Autodesk Inventor part; units mm, degrees
(part 3 of 6)
  arc A229 (-128.6396, 107.7295) -> (-129.027, 107.8036) centre (-130.0365, 101.4759) ccw projected
  arc A230 (-128.1665, 107.6078) -> (-128.6396, 107.7295) centre (-130.2936, 100.3247) ccw projected
  arc A231 (-128.1196, 107.2111) -> (-128.1665, 107.6078) centre (-148.5, 105) ccw projected
  arc A232 (-128.5511, 106.9822) -> (-128.1196, 107.2111) centre (-131.8881, 113.7963) ccw projected
  arc A233 (-128.9105, 106.8197) -> (-128.5511, 106.9822) centre (-131.3693, 112.7369) ccw projected
  arc A234 (-129.2005, 106.7091) -> (-128.9105, 106.8197) centre (-130.9335, 111.6881) ccw projected
  arc A235 (-129.1708, 106.331) -> (-129.2005, 106.7091) centre (-148.5, 105) ccw projected
  arc A236 (-128.867, 106.2671) -> (-129.1708, 106.331) centre (-130.1035, 101.1423) ccw projected
  arc A237 (-128.4867, 106.1629) -> (-128.867, 106.2671) centre (-130.3699, 100.0382) ccw projected
  arc A238 (-128.0246, 106.0044) -> (-128.4867, 106.1629) centre (-130.7166, 98.9106) ccw projected
  arc A239 (-128.0089, 105.6052) -> (-128.0246, 106.0044) centre (-148.5, 105) ccw projected
  arc A240 (-128.4571, 105.4109) -> (-128.0089, 105.6052) centre (-131.2492, 112.4658) ccw projected
  arc A241 (-128.8281, 105.2771) -> (-128.4571, 105.4109) centre (-130.8151, 111.369) ccw projected
  arc A242 (-129.1259, 105.1896) -> (-128.8281, 105.2771) centre (-130.4629, 110.2892) ccw projected
  arc A243 (-129.1259, 104.8104) -> (-129.1259, 105.1896) centre (-148.5, 105) ccw projected
  arc A244 (-128.8281, 104.7229) -> (-129.1259, 104.8104) centre (-130.4629, 99.7108) ccw projected
  arc A245 (-128.4571, 104.5891) -> (-128.8281, 104.7229) centre (-130.8151, 98.631) ccw projected
  arc A246 (-128.0089, 104.3948) -> (-128.4571, 104.5891) centre (-131.2492, 97.5342) ccw projected
  arc A247 (-128.0246, 103.9956) -> (-128.0089, 104.3948) centre (-148.5, 105) ccw projected
  arc A248 (-128.4867, 103.8371) -> (-128.0246, 103.9956) centre (-130.7166, 111.0894) ccw projected
  arc A249 (-128.867, 103.7329) -> (-128.4867, 103.8371) centre (-130.3699, 109.9618) ccw projected
  arc A250 (-129.1708, 103.669) -> (-128.867, 103.7329) centre (-130.1035, 108.8577) ccw projected
  arc A251 (-129.2005, 103.2909) -> (-129.1708, 103.669) centre (-148.5, 105) ccw projected
  arc A252 (-128.9105, 103.1803) -> (-129.2005, 103.2909) centre (-130.9335, 98.3119) ccw projected
  arc A253 (-128.5511, 103.0178) -> (-128.9105, 103.1803) centre (-131.3693, 97.2631) ccw projected
  arc A254 (-128.1196, 102.7889) -> (-128.5511, 103.0178) centre (-131.8881, 96.2037) ccw projected
  arc A255 (-128.1665, 102.3922) -> (-128.1196, 102.7889) centre (-148.5, 105) ccw projected
  arc A256 (-128.6396, 102.2705) -> (-128.1665, 102.3922) centre (-130.2936, 109.6753) ccw projected
  arc A257 (-129.027, 102.1964) -> (-128.6396, 102.2705) centre (-130.0365, 108.5241) ccw projected
  arc A258 (-129.3348, 102.1565) -> (-129.027, 102.1964) centre (-129.8575, 107.4025) ccw projected
  arc A259 (-129.3941, 101.7819) -> (-129.3348, 102.1565) centre (-148.5, 105) ccw projected
  arc A260 (-129.1137, 101.6489) -> (-129.3941, 101.7819) centre (-131.5124, 96.9543) ccw projected
  arc A261 (-128.7682, 101.4587) -> (-129.1137, 101.6489) centre (-132.0292, 95.9429) ccw projected
  arc A262 (-128.3559, 101.1967) -> (-128.7682, 101.4587) centre (-132.6295, 94.9274) ccw projected
  arc A263 (-128.4338, 100.8049) -> (-128.3559, 101.1967) centre (-148.5, 105) ccw projected
  arc A264 (-128.915, 100.7207) -> (-128.4338, 100.8049) centre (-129.983, 108.2324) ccw projected
  arc A265 (-129.307, 100.6772) -> (-128.915, 100.7207) centre (-129.8169, 107.0646) ccw projected
  arc A266 (-129.617, 100.6616) -> (-129.307, 100.6772) centre (-129.7265, 105.9324) ccw projected
  arc A267 (-129.7055, 100.2928) -> (-129.617, 100.6616) centre (-148.5, 105) ccw projected
  arc A268 (-129.4364, 100.1382) -> (-129.7055, 100.2928) centre (-132.196, 95.6463) ccw projected
  arc A269 (-129.1068, 99.9215) -> (-129.4364, 100.1382) centre (-132.7905, 94.6785) ccw projected
  arc A270 (-128.7164, 99.628) -> (-129.1068, 99.9215) centre (-133.4687, 93.7133) ccw projected
  arc A271 (-128.8248, 99.2435) -> (-128.7164, 99.628) centre (-148.5, 105) ccw projected
  arc A272 (-129.3111, 99.1972) -> (-128.8248, 99.2435) centre (-129.7864, 106.7696) ccw projected
  arc A273 (-129.7053, 99.1846) -> (-129.3111, 99.1972) centre (-129.7125, 105.5924) ccw projected
  arc A274 (-130.0156, 99.1934) -> (-129.7053, 99.1846) centre (-129.7112, 104.4566) ccw projected
  arc A275 (-130.1328, 98.8327) -> (-130.0156, 99.1934) centre (-148.5, 105) ccw projected
  arc A276 (-129.8766, 98.6575) -> (-130.1328, 98.8327) centre (-132.9801, 94.3959) ccw projected
  arc A277 (-129.5651, 98.4156) -> (-129.8766, 98.6575) centre (-133.6488, 93.4778) ccw projected
  arc A278 (-129.1989, 98.0923) -> (-129.5651, 98.4156) centre (-134.4006, 92.5688) ccw projected
  arc A279 (-129.3371, 97.7175) -> (-129.1989, 98.0923) centre (-148.5, 105) ccw projected
  arc A280 (-129.8255, 97.7096) -> (-129.3371, 97.7175) centre (-129.7053, 105.2959) ccw projected
  arc A281 (-130.2195, 97.728) -> (-129.8255, 97.7096) centre (-129.724, 104.1165) ccw projected
  arc A282 (-130.5281, 97.7611) -> (-130.2195, 97.728) centre (-129.8118, 102.9841) ccw projected
  arc A283 (-130.6733, 97.4107) -> (-130.5281, 97.7611) centre (-148.5, 105) ccw projected
  arc A284 (-130.4316, 97.2158) -> (-130.6733, 97.4107) centre (-133.86, 93.2109) ccw projected
  arc A285 (-130.14, 96.9503) -> (-130.4316, 97.2158) centre (-134.5986, 92.3481) ccw projected
  arc A286 (-129.8003, 96.5993) -> (-130.14, 96.9503) centre (-135.4194, 91.5009) ccw projected
  arc A287 (-129.9676, 96.2365) -> (-129.8003, 96.5993) centre (-148.5, 105) ccw projected
  arc A288 (-130.4551, 96.2669) -> (-129.9676, 96.2365) centre (-129.74, 103.8204) ccw projected
  arc A289 (-130.8464, 96.3161) -> (-130.4551, 96.2669) centre (-129.8512, 102.6461) ccw projected
  arc A290 (-131.1515, 96.3733) -> (-130.8464, 96.3161) centre (-130.0276, 101.524) ccw projected
  arc A291 (-131.3237, 96.0354) -> (-131.1515, 96.3733) centre (-148.5, 105) ccw projected
  arc A292 (-131.0981, 95.8222) -> (-131.3237, 96.0354) centre (-134.8301, 92.0986) ccw projected
  arc A293 (-130.8282, 95.5346) -> (-131.0981, 95.8222) centre (-135.6341, 91.2964) ccw projected
  arc A294 (-130.5171, 95.158) -> (-130.8282, 95.5346) centre (-136.5188, 90.5162) ccw projected
  arc A295 (-130.7123, 94.8095) -> (-130.5171, 95.158) centre (-148.5, 105) ccw projected
  arc A296 (-131.1959, 94.878) -> (-130.7123, 94.8095) centre (-129.8904, 102.3522) ccw projected
  arc A297 (-131.5822, 94.9578) -> (-131.1959, 94.878) centre (-130.0933, 101.1901) ccw projected
  arc A298 (-131.8818, 95.0388) -> (-131.5822, 94.9578) centre (-130.3572, 100.0854) ccw projected
  arc A299 (-132.08, 94.7154) -> (-131.8818, 95.0388) centre (-148.5, 105) ccw projected
  arc A300 (-131.8718, 94.4852) -> (-132.08, 94.7154) centre (-135.8844, 91.0659) ccw projected
  arc A301 (-131.6253, 94.1773) -> (-131.8718, 94.4852) centre (-136.7489, 90.3292) ccw projected
  arc A302 (-131.3447, 93.7774) -> (-131.6253, 94.1773) centre (-137.6922, 89.6208) ccw projected
  arc A303 (-131.5666, 93.4453) -> (-131.3447, 93.7774) centre (-148.5, 105) ccw projected
  arc A304 (-132.0434, 93.5515) -> (-131.5666, 93.4453) centre (-130.1555, 100.9002) ccw projected
  arc A305 (-132.4222, 93.6614) -> (-132.0434, 93.5515) centre (-130.449, 99.7577) ccw projected
  arc A306 (-132.7146, 93.7656) -> (-132.4222, 93.6614) centre (-130.7988, 98.6771) ccw projected
  arc A307 (-132.9375, 93.4588) -> (-132.7146, 93.7656) centre (-148.5, 105) ccw projected
  arc A308 (-132.748, 93.2129) -> (-132.9375, 93.4588) centre (-137.0166, 90.119) ccw projected
  arc A309 (-132.5265, 92.8866) -> (-132.748, 93.2129) centre (-137.9362, 89.4524) ccw projected
  arc A310 (-132.2781, 92.466) -> (-132.5265, 92.8866) centre (-138.9321, 88.8202) ccw projected
  arc A311 (-132.5254, 92.1523) -> (-132.2781, 92.466) centre (-148.5, 105) ccw projected
  arc A312 (-132.9924, 92.2957) -> (-132.5254, 92.1523) centre (-130.5337, 99.4736) ccw projected
  arc A313 (-133.3614, 92.4349) -> (-132.9924, 92.2957) centre (-130.9159, 98.3576) ccw projected
  arc A314 (-133.6447, 92.5617) -> (-133.3614, 92.4349) centre (-131.3494, 97.3078) ccw projected
  arc A315 (-133.891, 92.2734) -> (-133.6447, 92.5617) centre (-148.5, 105) ccw projected
  arc A316 (-133.7214, 92.0134) -> (-133.891, 92.2734) centre (-138.2195, 89.2639) ccw projected
  arc A317 (-133.5261, 91.6707) -> (-133.7214, 92.0134) centre (-139.1886, 88.6715) ccw projected
  arc A318 (-133.3115, 91.2319) -> (-133.5261, 91.6707) centre (-140.2311, 88.1194) ccw projected
  arc A319 (-133.5827, 90.9386) -> (-133.3115, 91.2319) centre (-148.5, 105) ccw projected
  arc A320 (-134.037, 91.1181) -> (-133.5827, 90.9386) centre (-131.0227, 98.081) ccw projected
  arc A321 (-134.3939, 91.2859) -> (-134.037, 91.1181) centre (-131.4913, 96.9985) ccw projected
  arc A322 (-134.6664, 91.4345) -> (-134.3939, 91.2859) centre (-132.0058, 95.9859) ccw projected
  arc A323 (-134.9345, 91.1664) -> (-134.6664, 91.4345) centre (-148.5, 105) ccw projected
  arc A324 (-134.7859, 90.8939) -> (-134.9345, 91.1664) centre (-139.4859, 88.5058) ccw projected
  arc A325 (-134.6181, 90.537) -> (-134.7859, 90.8939) centre (-140.4985, 87.9913) ccw projected
  arc A326 (-134.4386, 90.0827) -> (-134.6181, 90.537) centre (-141.581, 87.5227) ccw projected
  arc A327 (-134.7319, 89.8115) -> (-134.4386, 90.0827) centre (-148.5, 105) ccw projected
  arc A328 (-135.1707, 90.0261) -> (-134.7319, 89.8115) centre (-131.6194, 96.7311) ccw projected
  arc A329 (-135.5134, 90.2214) -> (-135.1707, 90.0261) centre (-132.1715, 95.6886) ccw projected
  arc A330 (-135.7734, 90.391) -> (-135.5134, 90.2214) centre (-132.7639, 94.7195) ccw projected
  arc A331 (-136.0617, 90.1447) -> (-135.7734, 90.391) centre (-148.5, 105) ccw projected
  arc A332 (-135.9349, 89.8614) -> (-136.0617, 90.1447) centre (-140.8078, 87.8494) ccw projected
  arc A333 (-135.7957, 89.4924) -> (-135.9349, 89.8614) centre (-141.8576, 87.4159) ccw projected
  arc A334 (-135.6523, 89.0254) -> (-135.7957, 89.4924) centre (-142.9736, 87.0337) ccw projected
  arc A335 (-135.966, 88.7781) -> (-135.6523, 89.0254) centre (-148.5, 105) ccw projected
  arc A336 (-136.3866, 89.0265) -> (-135.966, 88.7781) centre (-132.3202, 95.4321) ccw projected
  arc A337 (-136.7129, 89.248) -> (-136.3866, 89.0265) centre (-132.9524, 94.4362) ccw projected
  arc A338 (-136.9588, 89.4375) -> (-136.7129, 89.248) centre (-133.619, 93.5166) ccw projected
  arc A339 (-137.2656, 89.2146) -> (-136.9588, 89.4375) centre (-148.5, 105) ccw projected
  arc A340 (-137.1614, 88.9222) -> (-137.2656, 89.2146) centre (-142.1771, 87.2988) ccw projected
  arc A341 (-137.0515, 88.5434) -> (-137.1614, 88.9222) centre (-143.2577, 86.949) ccw projected
  arc A342 (-136.9453, 88.0666) -> (-137.0515, 88.5434) centre (-144.4002, 86.6555) ccw projected
  arc A343 (-137.2774, 87.8447) -> (-136.9453, 88.0666) centre (-148.5, 105) ccw projected
  arc A344 (-137.6773, 88.1253) -> (-137.2774, 87.8447) centre (-133.1208, 94.1922) ccw projected
  arc A345 (-137.9852, 88.3718) -> (-137.6773, 88.1253) centre (-133.8292, 93.2489) ccw projected
  arc A346 (-138.2154, 88.58) -> (-137.9852, 88.3718) centre (-134.5659, 92.3844) ccw projected
  arc A347 (-138.5388, 88.3818) -> (-138.2154, 88.58) centre (-148.5, 105) ccw projected
  arc A348 (-138.4578, 88.0822) -> (-138.5388, 88.3818) centre (-143.5854, 86.8572) ccw projected
  arc A349 (-138.378, 87.6959) -> (-138.4578, 88.0822) centre (-144.6901, 86.5933) ccw projected
  arc A350 (-138.3095, 87.2123) -> (-138.378, 87.6959) centre (-145.8522, 86.3904) ccw projected
  arc A351 (-138.658, 87.0171) -> (-138.3095, 87.2123) centre (-148.5, 105) ccw projected
  arc A352 (-139.0346, 87.3282) -> (-138.658, 87.0171) centre (-134.0162, 93.0188) ccw projected
  arc A353 (-139.3222, 87.5981) -> (-139.0346, 87.3282) centre (-134.7964, 92.1341) ccw projected
  arc A354 (-139.5354, 87.8237) -> (-139.3222, 87.5981) centre (-135.5986, 91.3301) ccw projected
  arc A355 (-139.8733, 87.6515) -> (-139.5354, 87.8237) centre (-148.5, 105) ccw projected
  arc A356 (-139.8161, 87.3464) -> (-139.8733, 87.6515) centre (-145.024, 86.5276) ccw projected
  arc A357 (-139.7669, 86.9551) -> (-139.8161, 87.3464) centre (-146.1461, 86.3512) ccw projected
  arc A358 (-139.7365, 86.4676) -> (-139.7669, 86.9551) centre (-147.3204, 86.24) ccw projected
  arc A359 (-140.0993, 86.3003) -> (-139.7365, 86.4676) centre (-148.5, 105) ccw projected
  arc A360 (-140.4503, 86.64) -> (-140.0993, 86.3003) centre (-135.0009, 91.9194) ccw projected
  arc A361 (-140.7158, 86.9316) -> (-140.4503, 86.64) centre (-135.8481, 91.0986) ccw projected
  arc A362 (-140.9107, 87.1733) -> (-140.7158, 86.9316) centre (-136.7109, 90.36) ccw projected
  arc A363 (-141.2611, 87.0281) -> (-140.9107, 87.1733) centre (-148.5, 105) ccw projected
  arc A364 (-141.228, 86.7195) -> (-141.2611, 87.0281) centre (-146.4841, 86.3118) ccw projected
  arc A365 (-141.2096, 86.3255) -> (-141.228, 86.7195) centre (-147.6165, 86.224) ccw projected
  arc A366 (-141.2175, 85.8371) -> (-141.2096, 86.3255) centre (-148.7959, 86.2053) ccw projected
  arc A367 (-141.5923, 85.6989) -> (-141.2175, 85.8371) centre (-148.5, 105) ccw projected
  arc A368 (-141.9156, 86.0651) -> (-141.5923, 85.6989) centre (-136.0688, 90.9006) ccw projected
  arc A369 (-142.1575, 86.3766) -> (-141.9156, 86.0651) centre (-136.9778, 90.1488) ccw projected
  arc A370 (-142.3327, 86.6328) -> (-142.1575, 86.3766) centre (-137.8959, 89.4801) ccw projected
  arc A371 (-142.6934, 86.5156) -> (-142.3327, 86.6328) centre (-148.5, 105) ccw projected
  arc A372 (-142.6846, 86.2053) -> (-142.6934, 86.5156) centre (-147.9566, 86.2112) ccw projected
  arc A373 (-142.6972, 85.8111) -> (-142.6846, 86.2053) centre (-149.0924, 86.2125) ccw projected
  arc A374 (-142.7435, 85.3248) -> (-142.6972, 85.8111) centre (-150.2696, 86.2864) ccw projected
  arc A375 (-143.128, 85.2164) -> (-142.7435, 85.3248) centre (-148.5, 105) ccw projected
  arc A376 (-143.4215, 85.6068) -> (-143.128, 85.2164) centre (-137.2133, 89.9687) ccw projected
  arc A377 (-143.6382, 85.9364) -> (-143.4215, 85.6068) centre (-138.1785, 89.2905) ccw projected
  arc A378 (-143.7928, 86.2055) -> (-143.6382, 85.9364) centre (-139.1463, 88.696) ccw projected
  arc A379 (-144.1616, 86.117) -> (-143.7928, 86.2055) centre (-148.5, 105) ccw projected
  arc A380 (-144.1772, 85.807) -> (-144.1616, 86.117) centre (-149.4324, 86.2265) ccw projected
  arc A381 (-144.2207, 85.415) -> (-144.1772, 85.807) centre (-150.5646, 86.3169) ccw projected
  arc A382 (-144.3049, 84.9338) -> (-144.2207, 85.415) centre (-151.7324, 86.483) ccw projected
  arc A383 (-144.6967, 84.8559) -> (-144.3049, 84.9338) centre (-148.5, 105) ccw projected
  arc A384 (-144.9587, 85.2682) -> (-144.6967, 84.8559) centre (-138.4274, 89.1295) ccw projected
  arc A385 (-145.1489, 85.6137) -> (-144.9587, 85.2682) centre (-139.4429, 88.5292) ccw projected
  arc A386 (-145.2819, 85.8941) -> (-145.1489, 85.6137) centre (-140.4543, 88.0124) ccw projected
  arc A387 (-145.6565, 85.8348) -> (-145.2819, 85.8941) centre (-148.5, 105) ccw projected
  arc A388 (-145.6964, 85.527) -> (-145.6565, 85.8348) centre (-150.9025, 86.3575) ccw projected
  arc A389 (-145.7705, 85.1396) -> (-145.6964, 85.527) centre (-152.0241, 86.5365) ccw projected
  arc A390 (-145.8922, 84.6665) -> (-145.7705, 85.1396) centre (-153.1753, 86.7936) ccw projected
  arc A391 (-146.2889, 84.6196) -> (-145.8922, 84.6665) centre (-148.5, 105) ccw projected
  arc A392 (-146.5178, 85.0511) -> (-146.2889, 84.6196) centre (-139.7037, 88.3881) ccw projected
  arc A393 (-146.6803, 85.4105) -> (-146.5178, 85.0511) centre (-140.7631, 87.8693) ccw projected
  arc A394 (-146.7909, 85.7005) -> (-146.6803, 85.4105) centre (-141.8119, 87.4335) ccw projected
  arc A395 (-147.169, 85.6708) -> (-146.7909, 85.7005) centre (-148.5, 105) ccw projected
  arc A396 (-147.2329, 85.367) -> (-147.169, 85.6708) centre (-152.3577, 86.6035) ccw projected
  arc A397 (-147.3371, 84.9867) -> (-147.2329, 85.367) centre (-153.4618, 86.8699) ccw projected
  arc A398 (-147.4956, 84.5246) -> (-147.3371, 84.9867) centre (-154.5894, 87.2166) ccw projected
  arc A399 (-147.8948, 84.5089) -> (-147.4956, 84.5246) centre (-148.5, 105) ccw projected
  arc A400 (-148.0891, 84.9571) -> (-147.8948, 84.5089) centre (-141.0342, 87.7492) ccw projected
  arc A401 (-148.2229, 85.3281) -> (-148.0891, 84.9571) centre (-142.131, 87.3151) ccw projected
  arc A402 (-148.3104, 85.6259) -> (-148.2229, 85.3281) centre (-143.2108, 86.9629) ccw projected
  arc A403 (-148.6896, 85.6259) -> (-148.3104, 85.6259) centre (-148.5, 105) ccw projected
  arc A404 (-148.7771, 85.3281) -> (-148.6896, 85.6259) centre (-153.7892, 86.9629) ccw projected
  arc A405 (-148.9109, 84.9571) -> (-148.7771, 85.3281) centre (-154.869, 87.3151) ccw projected
  arc A406 (-149.1052, 84.5089) -> (-148.9109, 84.9571) centre (-155.9658, 87.7492) ccw projected
  arc A407 (-149.5044, 84.5246) -> (-149.1052, 84.5089) centre (-148.5, 105) ccw projected
  arc A408 (-149.6629, 84.9867) -> (-149.5044, 84.5246) centre (-142.4106, 87.2166) ccw projected
  arc A409 (-149.7671, 85.367) -> (-149.6629, 84.9867) centre (-143.5382, 86.8699) ccw projected
  arc A410 (-149.831, 85.6708) -> (-149.7671, 85.367) centre (-144.6423, 86.6035) ccw projected
  arc A411 (-150.2091, 85.7005) -> (-149.831, 85.6708) centre (-148.5, 105) ccw projected
  arc A412 (-150.3197, 85.4105) -> (-150.2091, 85.7005) centre (-155.1881, 87.4335) ccw projected
  arc A413 (-150.4822, 85.0511) -> (-150.3197, 85.4105) centre (-156.2369, 87.8693) ccw projected
  arc A414 (-150.7111, 84.6196) -> (-150.4822, 85.0511) centre (-157.2963, 88.3881) ccw projected
  arc A415 (-151.1078, 84.6665) -> (-150.7111, 84.6196) centre (-148.5, 105) ccw projected
  arc A416 (-151.2295, 85.1396) -> (-151.1078, 84.6665) centre (-143.8247, 86.7936) ccw projected
  arc A417 (-151.3036, 85.527) -> (-151.2295, 85.1396) centre (-144.9759, 86.5365) ccw projected
  arc A418 (-151.3435, 85.8348) -> (-151.3036, 85.527) centre (-146.0975, 86.3575) ccw projected
  arc A419 (-151.7181, 85.8941) -> (-151.3435, 85.8348) centre (-148.5, 105) ccw projected
  arc A420 (-151.8511, 85.6137) -> (-151.7181, 85.8941) centre (-156.5457, 88.0124) ccw projected
  arc A421 (-152.0413, 85.2682) -> (-151.8511, 85.6137) centre (-157.5571, 88.5292) ccw projected
  arc A422 (-152.3033, 84.8559) -> (-152.0413, 85.2682) centre (-158.5726, 89.1295) ccw projected
  arc A423 (-152.6951, 84.9338) -> (-152.3033, 84.8559) centre (-148.5, 105) ccw projected
  arc A424 (-152.7793, 85.415) -> (-152.6951, 84.9338) centre (-145.2676, 86.483) ccw projected
  arc A425 (-152.8228, 85.807) -> (-152.7793, 85.415) centre (-146.4354, 86.3169) ccw projected
  arc A426 (-152.8384, 86.117) -> (-152.8228, 85.807) centre (-147.5676, 86.2265) ccw projected
  arc A427 (-153.2072, 86.2055) -> (-152.8384, 86.117) centre (-148.5, 105) ccw projected
  arc A428 (-153.3618, 85.9364) -> (-153.2072, 86.2055) centre (-157.8537, 88.696) ccw projected
  arc A429 (-153.5785, 85.6068) -> (-153.3618, 85.9364) centre (-158.8215, 89.2905) ccw projected
  arc A430 (-153.872, 85.2164) -> (-153.5785, 85.6068) centre (-159.7867, 89.9687) ccw projected
  arc A431 (-154.2565, 85.3248) -> (-153.872, 85.2164) centre (-148.5, 105) ccw projected
  arc A432 (-154.3028, 85.8111) -> (-154.2565, 85.3248) centre (-146.7304, 86.2864) ccw projected
  arc A433 (-154.3154, 86.2053) -> (-154.3028, 85.8111) centre (-147.9076, 86.2125) ccw projected
  arc A434 (-154.3066, 86.5156) -> (-154.3154, 86.2053) centre (-149.0434, 86.2112) ccw projected
  arc A435 (-154.6673, 86.6328) -> (-154.3066, 86.5156) centre (-148.5, 105) ccw projected
  arc A436 (-154.8425, 86.3766) -> (-154.6673, 86.6328) centre (-159.1041, 89.4801) ccw projected
  arc A437 (-155.0844, 86.0651) -> (-154.8425, 86.3766) centre (-160.0222, 90.1488) ccw projected
  arc A438 (-155.4077, 85.6989) -> (-155.0844, 86.0651) centre (-160.9312, 90.9006) ccw projected
  arc A439 (-155.7825, 85.8371) -> (-155.4077, 85.6989) centre (-148.5, 105) ccw projected
  arc A440 (-155.7904, 86.3255) -> (-155.7825, 85.8371) centre (-148.2041, 86.2053) ccw projected
  arc A441 (-155.772, 86.7195) -> (-155.7904, 86.3255) centre (-149.3835, 86.224) ccw projected
  arc A442 (-155.7389, 87.0281) -> (-155.772, 86.7195) centre (-150.5159, 86.3118) ccw projected
  arc A443 (-156.0893, 87.1733) -> (-155.7389, 87.0281) centre (-148.5, 105) ccw projected
  arc A444 (-156.2842, 86.9316) -> (-156.0893, 87.1733) centre (-160.2891, 90.36) ccw projected
  arc A445 (-156.5497, 86.64) -> (-156.2842, 86.9316) centre (-161.1519, 91.0986) ccw projected
  arc A446 (-156.9007, 86.3003) -> (-156.5497, 86.64) centre (-161.9991, 91.9194) ccw projected
  arc A447 (-157.2635, 86.4676) -> (-156.9007, 86.3003) centre (-148.5, 105) ccw projected
  arc A448 (-157.2331, 86.9551) -> (-157.2635, 86.4676) centre (-149.6796, 86.24) ccw projected
  arc A449 (-157.1839, 87.3464) -> (-157.2331, 86.9551) centre (-150.8539, 86.3512) ccw projected
  arc A450 (-157.1267, 87.6515) -> (-157.1839, 87.3464) centre (-151.976, 86.5276) ccw projected
  arc A451 (-157.4646, 87.8237) -> (-157.1267, 87.6515) centre (-148.5, 105) ccw projected
  arc A452 (-157.6778, 87.5981) -> (-157.4646, 87.8237) centre (-161.4014, 91.3301) ccw projected
  arc A453 (-157.9654, 87.3282) -> (-157.6778, 87.5981) centre (-162.2036, 92.1341) ccw projected
  arc A454 (-158.342, 87.0171) -> (-157.9654, 87.3282) centre (-162.9838, 93.0188) ccw projected
  arc A455 (-158.6905, 87.2123) -> (-158.342, 87.0171) centre (-148.5, 105) ccw projected
  arc A456 (-158.622, 87.6959) -> (-158.6905, 87.2123) centre (-151.1478, 86.3904) ccw projected
  arc A457 (-158.5422, 88.0822) -> (-158.622, 87.6959) centre (-152.3099, 86.5933) ccw projected
  arc A458 (-158.4612, 88.3818) -> (-158.5422, 88.0822) centre (-153.4146, 86.8572) ccw projected
  arc A459 (-158.7846, 88.58) -> (-158.4612, 88.3818) centre (-148.5, 105) ccw projected
  arc A460 (-159.0148, 88.3718) -> (-158.7846, 88.58) centre (-162.4341, 92.3844) ccw projected
  arc A461 (-159.3227, 88.1253) -> (-159.0148, 88.3718) centre (-163.1708, 93.2489) ccw projected
  arc A462 (-159.7226, 87.8447) -> (-159.3227, 88.1253) centre (-163.8792, 94.1922) ccw projected
  arc A463 (-160.0547, 88.0666) -> (-159.7226, 87.8447) centre (-148.5, 105) ccw projected
  arc A464 (-159.9485, 88.5434) -> (-160.0547, 88.0666) centre (-152.5998, 86.6555) ccw projected
  arc A465 (-159.8386, 88.9222) -> (-159.9485, 88.5434) centre (-153.7423, 86.949) ccw projected
  arc A466 (-159.7344, 89.2146) -> (-159.8386, 88.9222) centre (-154.8229, 87.2988) ccw projected
  arc A467 (-160.0412, 89.4375) -> (-159.7344, 89.2146) centre (-148.5, 105) ccw projected
  arc A468 (-160.2871, 89.248) -> (-160.0412, 89.4375) centre (-163.381, 93.5166) ccw projected
  arc A469 (-160.6134, 89.0265) -> (-160.2871, 89.248) centre (-164.0476, 94.4362) ccw projected
  arc A470 (-161.034, 88.7781) -> (-160.6134, 89.0265) centre (-164.6798, 95.4321) ccw projected
  arc A471 (-161.3477, 89.0254) -> (-161.034, 88.7781) centre (-148.5, 105) ccw projected
  arc A472 (-161.2043, 89.4924) -> (-161.3477, 89.0254) centre (-154.0264, 87.0337) ccw projected
  arc A473 (-161.0651, 89.8614) -> (-161.2043, 89.4924) centre (-155.1424, 87.4159) ccw projected
  arc A474 (-160.9383, 90.1447) -> (-161.0651, 89.8614) centre (-156.1922, 87.8494) ccw projected
  arc A475 (-161.2266, 90.391) -> (-160.9383, 90.1447) centre (-148.5, 105) ccw projected
  arc A476 (-161.4866, 90.2214) -> (-161.2266, 90.391) centre (-164.2361, 94.7195) ccw projected
  arc A477 (-161.8293, 90.0261) -> (-161.4866, 90.2214) centre (-164.8285, 95.6886) ccw projected
  arc A478 (-162.2681, 89.8115) -> (-161.8293, 90.0261) centre (-165.3806, 96.7311) ccw projected
  arc A479 (-162.5614, 90.0827) -> (-162.2681, 89.8115) centre (-148.5, 105) ccw projected
  arc A480 (-162.3819, 90.537) -> (-162.5614, 90.0827) centre (-155.419, 87.5227) ccw projected
  arc A481 (-162.2141, 90.8939) -> (-162.3819, 90.537) centre (-156.5015, 87.9913) ccw projected
  arc A482 (-162.0655, 91.1664) -> (-162.2141, 90.8939) centre (-157.5141, 88.5058) ccw projected
  arc A483 (-162.3336, 91.4345) -> (-162.0655, 91.1664) centre (-148.5, 105) ccw projected
  arc A484 (-162.6061, 91.2859) -> (-162.3336, 91.4345) centre (-164.9942, 95.9859) ccw projected
  arc A485 (-162.963, 91.1181) -> (-162.6061, 91.2859) centre (-165.5087, 96.9985) ccw projected
  arc A486 (-163.4173, 90.9386) -> (-162.963, 91.1181) centre (-165.9773, 98.081) ccw projected
  arc A487 (-163.6885, 91.2319) -> (-163.4173, 90.9386) centre (-148.5, 105) ccw projected
  arc A488 (-163.4738, 91.6707) -> (-163.6885, 91.2319) centre (-156.7689, 88.1194) ccw projected
  arc A489 (-163.2786, 92.0134) -> (-163.4738, 91.6707) centre (-157.8114, 88.6715) ccw projected
  arc A490 (-163.109, 92.2734) -> (-163.2786, 92.0134) centre (-158.7805, 89.2639) ccw projected
  arc A491 (-163.3553, 92.5617) -> (-163.109, 92.2734) centre (-148.5, 105) ccw projected
  arc A492 (-163.6386, 92.4349) -> (-163.3553, 92.5617) centre (-165.6506, 97.3078) ccw projected
  arc A493 (-164.0076, 92.2957) -> (-163.6386, 92.4349) centre (-166.0841, 98.3576) ccw projected
  arc A494 (-164.4746, 92.1523) -> (-164.0076, 92.2957) centre (-166.4663, 99.4736) ccw projected
  arc A495 (-164.7219, 92.466) -> (-164.4746, 92.1523) centre (-148.5, 105) ccw projected
  arc A496 (-164.4735, 92.8866) -> (-164.7219, 92.466) centre (-158.0679, 88.8202) ccw projected
  arc A497 (-164.252, 93.2129) -> (-164.4735, 92.8866) centre (-159.0638, 89.4524) ccw projected
  arc A498 (-164.0625, 93.4588) -> (-164.252, 93.2129) centre (-159.9834, 90.119) ccw projected
  arc A499 (-164.2854, 93.7656) -> (-164.0625, 93.4588) centre (-148.5, 105) ccw projected
  arc A500 (-164.5778, 93.6614) -> (-164.2854, 93.7656) centre (-166.2012, 98.6771) ccw projected
  arc A501 (-164.9566, 93.5515) -> (-164.5778, 93.6614) centre (-166.551, 99.7577) ccw projected
  arc A502 (-165.4334, 93.4453) -> (-164.9566, 93.5515) centre (-166.8445, 100.9002) ccw projected
  arc A503 (-165.6553, 93.7774) -> (-165.4334, 93.4453) centre (-148.5, 105) ccw projected
  arc A504 (-165.3747, 94.1773) -> (-165.6553, 93.7774) centre (-159.3078, 89.6208) ccw projected
  arc A505 (-165.1282, 94.4852) -> (-165.3747, 94.1773) centre (-160.2511, 90.3292) ccw projected
  arc A506 (-164.92, 94.7154) -> (-165.1282, 94.4852) centre (-161.1156, 91.0659) ccw projected
  arc A507 (-165.1182, 95.0388) -> (-164.92, 94.7154) centre (-148.5, 105) ccw projected
  arc A508 (-165.4178, 94.9578) -> (-165.1182, 95.0388) centre (-166.6428, 100.0854) ccw projected
  arc A509 (-165.8041, 94.878) -> (-165.4178, 94.9578) centre (-166.9067, 101.1901) ccw projected
  arc A510 (-166.2877, 94.8095) -> (-165.8041, 94.878) centre (-167.1096, 102.3522) ccw projected
  arc A511 (-166.4829, 95.158) -> (-166.2877, 94.8095) centre (-148.5, 105) ccw projected
  arc A512 (-166.1718, 95.5346) -> (-166.4829, 95.158) centre (-160.4812, 90.5162) ccw projected
  arc A513 (-165.9019, 95.8222) -> (-166.1718, 95.5346) centre (-161.3659, 91.2964) ccw projected
  arc A514 (-165.6763, 96.0354) -> (-165.9019, 95.8222) centre (-162.1699, 92.0986) ccw projected
  arc A515 (-165.8485, 96.3733) -> (-165.6763, 96.0354) centre (-148.5, 105) ccw projected
  arc A516 (-166.1536, 96.3161) -> (-165.8485, 96.3733) centre (-166.9724, 101.524) ccw projected
  arc A517 (-166.5449, 96.2669) -> (-166.1536, 96.3161) centre (-167.1488, 102.6461) ccw projected
  arc A518 (-167.0324, 96.2365) -> (-166.5449, 96.2669) centre (-167.26, 103.8204) ccw projected
  arc A519 (-167.1997, 96.5993) -> (-167.0324, 96.2365) centre (-148.5, 105) ccw projected
  arc A520 (-166.86, 96.9503) -> (-167.1997, 96.5993) centre (-161.5806, 91.5009) ccw projected
  arc A521 (-166.5684, 97.2158) -> (-166.86, 96.9503) centre (-162.4014, 92.3481) ccw projected
  arc A522 (-166.3267, 97.4107) -> (-166.5684, 97.2158) centre (-163.14, 93.2109) ccw projected
  arc A523 (-166.4719, 97.7611) -> (-166.3267, 97.4107) centre (-148.5, 105) ccw projected
  arc A524 (-166.7805, 97.728) -> (-166.4719, 97.7611) centre (-167.1882, 102.9841) ccw projected
  arc A525 (-167.1745, 97.7096) -> (-166.7805, 97.728) centre (-167.276, 104.1165) ccw projected
  arc A526 (-167.6629, 97.7175) -> (-167.1745, 97.7096) centre (-167.2947, 105.2959) ccw projected
  arc A527 (-167.8011, 98.0923) -> (-167.6629, 97.7175) centre (-148.5, 105) ccw projected
  arc A528 (-167.4349, 98.4156) -> (-167.8011, 98.0923) centre (-162.5994, 92.5688) ccw projected
  arc A529 (-167.1234, 98.6575) -> (-167.4349, 98.4156) centre (-163.3512, 93.4778) ccw projected
  arc A530 (-166.8672, 98.8327) -> (-167.1234, 98.6575) centre (-164.0199, 94.3959) ccw projected
  arc A531 (-166.9844, 99.1934) -> (-166.8672, 98.8327) centre (-148.5, 105) ccw projected
  arc A532 (-167.2947, 99.1846) -> (-166.9844, 99.1934) centre (-167.2888, 104.4566) ccw projected
  arc A533 (-167.6889, 99.1972) -> (-167.2947, 99.1846) centre (-167.2875, 105.5924) ccw projected
  arc A534 (-168.1752, 99.2435) -> (-167.6889, 99.1972) centre (-167.2136, 106.7696) ccw projected
  arc A535 (-168.2836, 99.628) -> (-168.1752, 99.2435) centre (-148.5, 105) ccw projected
  arc A536 (-167.8932, 99.9215) -> (-168.2836, 99.628) centre (-163.5313, 93.7133) ccw projected
  arc A537 (-167.5636, 100.1382) -> (-167.8932, 99.9215) centre (-164.2095, 94.6785) ccw projected
  arc A538 (-167.2945, 100.2928) -> (-167.5636, 100.1382) centre (-164.804, 95.6463) ccw projected
  arc A539 (-167.383, 100.6616) -> (-167.2945, 100.2928) centre (-148.5, 105) ccw projected
  arc A540 (-167.693, 100.6772) -> (-167.383, 100.6616) centre (-167.2735, 105.9324) ccw projected
  arc A541 (-168.085, 100.7207) -> (-167.693, 100.6772) centre (-167.1831, 107.0646) ccw projected
  arc A542 (-168.5662, 100.8049) -> (-168.085, 100.7207) centre (-167.017, 108.2324) ccw projected
  arc A543 (-168.6441, 101.1967) -> (-168.5662, 100.8049) centre (-148.5, 105) ccw projected
  arc A544 (-168.2318, 101.4587) -> (-168.6441, 101.1967) centre (-164.3705, 94.9274) ccw projected
  arc A545 (-167.8863, 101.6489) -> (-168.2318, 101.4587) centre (-164.9708, 95.9429) ccw projected
  arc A546 (-167.6059, 101.7819) -> (-167.8863, 101.6489) centre (-165.4876, 96.9543) ccw projected
  arc A547 (-167.6652, 102.1565) -> (-167.6059, 101.7819) centre (-148.5, 105) ccw projected
  arc A548 (-167.973, 102.1964) -> (-167.6652, 102.1565) centre (-167.1425, 107.4025) ccw projected
  arc A549 (-168.3604, 102.2705) -> (-167.973, 102.1964) centre (-166.9635, 108.5241) ccw projected
  arc A550 (-168.8335, 102.3922) -> (-168.3604, 102.2705) centre (-166.7064, 109.6753) ccw projected
  arc A551 (-168.8804, 102.7889) -> (-168.8335, 102.3922) centre (-148.5, 105) ccw projected
  arc A552 (-168.4489, 103.0178) -> (-168.8804, 102.7889) centre (-165.1119, 96.2037) ccw projected
  arc A553 (-168.0895, 103.1803) -> (-168.4489, 103.0178) centre (-165.6307, 97.2631) ccw projected
  arc A554 (-167.7995, 103.2909) -> (-168.0895, 103.1803) centre (-166.0665, 98.3119) ccw projected
  arc A555 (-167.8292, 103.669) -> (-167.7995, 103.2909) centre (-148.5, 105) ccw projected
  arc A556 (-168.133, 103.7329) -> (-167.8292, 103.669) centre (-166.8965, 108.8577) ccw projected
  arc A557 (-168.5133, 103.8371) -> (-168.133, 103.7329) centre (-166.6301, 109.9618) ccw projected
  arc A558 (-168.9754, 103.9956) -> (-168.5133, 103.8371) centre (-166.2834, 111.0894) ccw projected
  arc A559 (-168.9911, 104.3948) -> (-168.9754, 103.9956) centre (-148.5, 105) ccw projected
  arc A560 (-168.5429, 104.5891) -> (-168.9911, 104.3948) centre (-165.7508, 97.5342) ccw projected
  arc A561 (-168.1719, 104.7229) -> (-168.5429, 104.5891) centre (-166.1849, 98.631) ccw projected
  arc A562 (-167.8741, 104.8104) -> (-168.1719, 104.7229) centre (-166.5371, 99.7108) ccw projected
  arc A563 (-167.8741, 105.1896) -> (-167.8741, 104.8104) centre (-148.5, 105) ccw projected
  arc A564 (-168.1719, 105.2771) -> (-167.8741, 105.1896) centre (-166.5371, 110.2892) ccw projected
  arc A565 (-168.5429, 105.4109) -> (-168.1719, 105.2771) centre (-166.1849, 111.369) ccw projected
  arc A566 (-168.9911, 105.6052) -> (-168.5429, 105.4109) centre (-165.7508, 112.4658) ccw projected
  arc A567 (-168.9754, 106.0044) -> (-168.9911, 105.6052) centre (-148.5, 105) ccw projected
  arc A568 (-168.5133, 106.1629) -> (-168.9754, 106.0044) centre (-166.2834, 98.9106) ccw projected
  arc A569 (-168.133, 106.2671) -> (-168.5133, 106.1629) centre (-166.6301, 100.0382) ccw projected
  arc A570 (-167.8292, 106.331) -> (-168.133, 106.2671) centre (-166.8965, 101.1423) ccw projected
  arc A571 (-167.7995, 106.7091) -> (-167.8292, 106.331) centre (-148.5, 105) ccw projected
  arc A572 (-168.0895, 106.8197) -> (-167.7995, 106.7091) centre (-166.0665, 111.6881) ccw projected
  arc A573 (-168.4489, 106.9822) -> (-168.0895, 106.8197) centre (-165.6307, 112.7369) ccw projected
  arc A574 (-168.8804, 107.2111) -> (-168.4489, 106.9822) centre (-165.1119, 113.7963) ccw projected
  arc A575 (-168.8335, 107.6078) -> (-168.8804, 107.2111) centre (-148.5, 105) ccw projected
  arc A576 (-168.3604, 107.7295) -> (-168.8335, 107.6078) centre (-166.7064, 100.3247) ccw projected
  arc A577 (-167.973, 107.8036) -> (-168.3604, 107.7295) centre (-166.9635, 101.4759) ccw projected
  arc A578 (-167.6652, 107.8435) -> (-167.973, 107.8036) centre (-167.1425, 102.5975) ccw projected
  arc A579 (-167.6059, 108.2181) -> (-167.6652, 107.8435) centre (-148.5, 105) ccw projected
  arc A580 (-167.8863, 108.3511) -> (-167.6059, 108.2181) centre (-165.4876, 113.0457) ccw projected
  arc A581 (-168.2318, 108.5413) -> (-167.8863, 108.3511) centre (-164.9708, 114.0571) ccw projected
  arc A582 (-168.6441, 108.8033) -> (-168.2318, 108.5413) centre (-164.3705, 115.0726) ccw projected
  arc A583 (-168.5662, 109.1951) -> (-168.6441, 108.8033) centre (-148.5, 105) ccw projected
  arc A584 (-168.085, 109.2793) -> (-168.5662, 109.1951) centre (-167.017, 101.7676) ccw projected
  arc A585 (-167.693, 109.3228) -> (-168.085, 109.2793) centre (-167.1831, 102.9354) ccw projected
  arc A586 (-167.383, 109.3384) -> (-167.693, 109.3228) centre (-167.2735, 104.0676) ccw projected
  arc A587 (-167.2945, 109.7072) -> (-167.383, 109.3384) centre (-148.5, 105) ccw projected
  arc A588 (-167.5636, 109.8618) -> (-167.2945, 109.7072) centre (-164.804, 114.3537) ccw projected
  arc A589 (-167.8932, 110.0785) -> (-167.5636, 109.8618) centre (-164.2095, 115.3215) ccw projected
  arc A590 (-168.2836, 110.372) -> (-167.8932, 110.0785) centre (-163.5313, 116.2867) ccw projected
  arc A591 (-168.1752, 110.7565) -> (-168.2836, 110.372) centre (-148.5, 105) ccw projected
  arc A592 (-167.6889, 110.8028) -> (-168.1752, 110.7565) centre (-167.2136, 103.2304) ccw projected
  arc A593 (-167.2947, 110.8154) -> (-167.6889, 110.8028) centre (-167.2875, 104.4076) ccw projected
  arc A594 (-166.9844, 110.8066) -> (-167.2947, 110.8154) centre (-167.2888, 105.5434) ccw projected
  arc A595 (-166.8672, 111.1673) -> (-166.9844, 110.8066) centre (-148.5, 105) ccw projected
  arc A596 (-167.1234, 111.3425) -> (-166.8672, 111.1673) centre (-164.0199, 115.6041) ccw projected
  arc A597 (-167.4349, 111.5844) -> (-167.1234, 111.3425) centre (-163.3512, 116.5222) ccw projected
  arc A598 (-167.8011, 111.9077) -> (-167.4349, 111.5844) centre (-162.5994, 117.4312) ccw projected
  arc A599 (-167.6629, 112.2825) -> (-167.8011, 111.9077) centre (-148.5, 105) ccw projected
  arc A600 (-167.1745, 112.2904) -> (-167.6629, 112.2825) centre (-167.2947, 104.7041) ccw projected
  arc A601 (-166.7805, 112.272) -> (-167.1745, 112.2904) centre (-167.276, 105.8835) ccw projected
  arc A602 (-166.4719, 112.2389) -> (-166.7805, 112.272) centre (-167.1882, 107.0159) ccw projected
  arc A603 (-166.3267, 112.5893) -> (-166.4719, 112.2389) centre (-148.5, 105) ccw projected
  arc A604 (-166.5684, 112.7842) -> (-166.3267, 112.5893) centre (-163.14, 116.7891) ccw projected
  arc A605 (-166.86, 113.0497) -> (-166.5684, 112.7842) centre (-162.4014, 117.6519) ccw projected
  arc A606 (-167.1997, 113.4007) -> (-166.86, 113.0497) centre (-161.5806, 118.4991) ccw projected
  arc A607 (-167.0324, 113.7635) -> (-167.1997, 113.4007) centre (-148.5, 105) ccw projected
  arc A608 (-166.5449, 113.7331) -> (-167.0324, 113.7635) centre (-167.26, 106.1796) ccw projected
  arc A609 (-166.1536, 113.6839) -> (-166.5449, 113.7331) centre (-167.1488, 107.3539) ccw projected
  arc A610 (-165.8485, 113.6267) -> (-166.1536, 113.6839) centre (-166.9724, 108.476) ccw projected
  arc A611 (-165.6763, 113.9646) -> (-165.8485, 113.6267) centre (-148.5, 105) ccw projected
  arc A612 (-165.9019, 114.1778) -> (-165.6763, 113.9646) centre (-162.1699, 117.9014) ccw projected
  arc A613 (-166.1718, 114.4654) -> (-165.9019, 114.1778) centre (-161.3659, 118.7036) ccw projected
  arc A614 (-166.4829, 114.842) -> (-166.1718, 114.4654) centre (-160.4812, 119.4838) ccw projected
  arc A615 (-166.2877, 115.1905) -> (-166.4829, 114.842) centre (-148.5, 105) ccw projected
  arc A616 (-165.8041, 115.122) -> (-166.2877, 115.1905) centre (-167.1096, 107.6478) ccw projected
  arc A617 (-165.4178, 115.0422) -> (-165.8041, 115.122) centre (-166.9067, 108.8099) ccw projected
  arc A618 (-165.1182, 114.9612) -> (-165.4178, 115.0422) centre (-166.6428, 109.9146) ccw projected
  arc A619 (-164.92, 115.2846) -> (-165.1182, 114.9612) centre (-148.5, 105) ccw projected
  arc A620 (-165.1282, 115.5148) -> (-164.92, 115.2846) centre (-161.1156, 118.9341) ccw projected
  arc A621 (-165.3747, 115.8227) -> (-165.1282, 115.5148) centre (-160.2511, 119.6708) ccw projected
  arc A622 (-165.6553, 116.2226) -> (-165.3747, 115.8227) centre (-159.3078, 120.3792) ccw projected
  arc A623 (-165.4334, 116.5547) -> (-165.6553, 116.2226) centre (-148.5, 105) ccw projected
  arc A624 (-164.9566, 116.4485) -> (-165.4334, 116.5547) centre (-166.8445, 109.0998) ccw projected
  arc A625 (-164.5778, 116.3386) -> (-164.9566, 116.4485) centre (-166.551, 110.2423) ccw projected
  arc A626 (-164.2854, 116.2344) -> (-164.5778, 116.3386) centre (-166.2012, 111.3229) ccw projected
  arc A627 (-164.0625, 116.5412) -> (-164.2854, 116.2344) centre (-148.5, 105) ccw projected
  arc A628 (-164.252, 116.7871) -> (-164.0625, 116.5412) centre (-159.9834, 119.881) ccw projected
  arc A629 (-164.4735, 117.1134) -> (-164.252, 116.7871) centre (-159.0638, 120.5476) ccw projected
  arc A630 (-164.7219, 117.534) -> (-164.4735, 117.1134) centre (-158.0679, 121.1798) ccw projected
  arc A631 (-164.4746, 117.8477) -> (-164.7219, 117.534) centre (-148.5, 105) ccw projected
  arc A632 (-164.0076, 117.7043) -> (-164.4746, 117.8477) centre (-166.4663, 110.5264) ccw projected
  arc A633 (-163.6386, 117.5651) -> (-164.0076, 117.7043) centre (-166.0841, 111.6424) ccw projected
  arc A634 (-163.3553, 117.4383) -> (-163.6386, 117.5651) centre (-165.6506, 112.6922) ccw projected
  arc A635 (-163.109, 117.7266) -> (-163.3553, 117.4383) centre (-148.5, 105) ccw projected
  arc A636 (-163.2786, 117.9866) -> (-163.109, 117.7266) centre (-158.7805, 120.7361) ccw projected
  arc A637 (-163.4738, 118.3293) -> (-163.2786, 117.9866) centre (-157.8114, 121.3285) ccw projected
  arc A638 (-163.6885, 118.7681) -> (-163.4738, 118.3293) centre (-156.7689, 121.8806) ccw projected
  arc A639 (-163.4173, 119.0614) -> (-163.6885, 118.7681) centre (-148.5, 105) ccw projected
  arc A640 (-162.963, 118.8819) -> (-163.4173, 119.0614) centre (-165.9773, 111.919) ccw projected
  arc A641 (-162.6061, 118.7141) -> (-162.963, 118.8819) centre (-165.5087, 113.0015) ccw projected
  arc A642 (-162.3336, 118.5655) -> (-162.6061, 118.7141) centre (-164.9942, 114.0141) ccw projected
  arc A643 (-162.0655, 118.8336) -> (-162.3336, 118.5655) centre (-148.5, 105) ccw projected
  arc A644 (-162.2141, 119.1061) -> (-162.0655, 118.8336) centre (-157.5141, 121.4942) ccw projected
  arc A645 (-162.3819, 119.463) -> (-162.2141, 119.1061) centre (-156.5015, 122.0087) ccw projected
  arc A646 (-162.5614, 119.9173) -> (-162.3819, 119.463) centre (-155.419, 122.4773) ccw projected
  arc A647 (-162.2681, 120.1885) -> (-162.5614, 119.9173) centre (-148.5, 105) ccw projected
  arc A648 (-161.8293, 119.9739) -> (-162.2681, 120.1885) centre (-165.3806, 113.2689) ccw projected
  arc A649 (-161.4866, 119.7786) -> (-161.8293, 119.9739) centre (-164.8285, 114.3114) ccw projected
  arc A650 (-161.2266, 119.609) -> (-161.4866, 119.7786) centre (-164.2361, 115.2805) ccw projected
  arc A651 (-160.9383, 119.8553) -> (-161.2266, 119.609) centre (-148.5, 105) ccw projected
  arc A652 (-161.0651, 120.1386) -> (-160.9383, 119.8553) centre (-156.1922, 122.1506) ccw projected
  arc A653 (-161.2043, 120.5076) -> (-161.0651, 120.1386) centre (-155.1424, 122.5841) ccw projected
  arc A654 (-161.3477, 120.9746) -> (-161.2043, 120.5076) centre (-154.0264, 122.9663) ccw projected
  arc A655 (-161.034, 121.2219) -> (-161.3477, 120.9746) centre (-148.5, 105) ccw projected
  arc A656 (-160.6134, 120.9735) -> (-161.034, 121.2219) centre (-164.6798, 114.5679) ccw projected
  arc A657 (-160.2871, 120.752) -> (-160.6134, 120.9735) centre (-164.0476, 115.5638) ccw projected
  arc A658 (-160.0412, 120.5625) -> (-160.2871, 120.752) centre (-163.381, 116.4834) ccw projected
  arc A659 (-159.7344, 120.7854) -> (-160.0412, 120.5625) centre (-148.5, 105) ccw projected
  arc A660 (-159.8386, 121.0778) -> (-159.7344, 120.7854) centre (-154.8229, 122.7012) ccw projected
  arc A661 (-159.9485, 121.4566) -> (-159.8386, 121.0778) centre (-153.7423, 123.051) ccw projected
  arc A662 (-160.0547, 121.9334) -> (-159.9485, 121.4566) centre (-152.5998, 123.3445) ccw projected
  arc A663 (-159.7226, 122.1553) -> (-160.0547, 121.9334) centre (-148.5, 105) ccw projected
  arc A664 (-159.3227, 121.8747) -> (-159.7226, 122.1553) centre (-163.8792, 115.8078) ccw projected
  arc A665 (-159.0148, 121.6282) -> (-159.3227, 121.8747) centre (-163.1708, 116.7511) ccw projected
  arc A666 (-158.7846, 121.42) -> (-159.0148, 121.6282) centre (-162.4341, 117.6156) ccw projected
  arc A667 (-158.4612, 121.6182) -> (-158.7846, 121.42) centre (-148.5, 105) ccw projected
  arc A668 (-158.5422, 121.9178) -> (-158.4612, 121.6182) centre (-153.4146, 123.1428) ccw projected
  arc A669 (-158.622, 122.3041) -> (-158.5422, 121.9178) centre (-152.3099, 123.4067) ccw projected
  arc A670 (-158.6905, 122.7877) -> (-158.622, 122.3041) centre (-151.1478, 123.6096) ccw projected
  arc A671 (-158.342, 122.9829) -> (-158.6905, 122.7877) centre (-148.5, 105) ccw projected
  arc A672 (-157.9654, 122.6718) -> (-158.342, 122.9829) centre (-162.9838, 116.9812) ccw projected
  arc A673 (-157.6778, 122.4019) -> (-157.9654, 122.6718) centre (-162.2036, 117.8659) ccw projected
  arc A674 (-157.4646, 122.1763) -> (-157.6778, 122.4019) centre (-161.4014, 118.6699) ccw projected
  arc A675 (-157.1267, 122.3485) -> (-157.4646, 122.1763) centre (-148.5, 105) ccw projected
  arc A676 (-157.1839, 122.6536) -> (-157.1267, 122.3485) centre (-151.976, 123.4724) ccw projected
  arc A677 (-157.2331, 123.0449) -> (-157.1839, 122.6536) centre (-150.8539, 123.6488) ccw projected
  arc A678 (-157.2635, 123.5324) -> (-157.2331, 123.0449) centre (-149.6796, 123.76) ccw projected
  arc A679 (-156.9007, 123.6997) -> (-157.2635, 123.5324) centre (-148.5, 105) ccw projected
  arc A680 (-156.5497, 123.36) -> (-156.9007, 123.6997) centre (-161.9991, 118.0806) ccw projected
  arc A681 (-156.2842, 123.0684) -> (-156.5497, 123.36) centre (-161.1519, 118.9014) ccw projected
  arc A682 (-156.0893, 122.8267) -> (-156.2842, 123.0684) centre (-160.2891, 119.64) ccw projected
  arc A683 (-155.7389, 122.9719) -> (-156.0893, 122.8267) centre (-148.5, 105) ccw projected
  arc A684 (-155.772, 123.2805) -> (-155.7389, 122.9719) centre (-150.5159, 123.6882) ccw projected
  arc A685 (-155.7904, 123.6745) -> (-155.772, 123.2805) centre (-149.3835, 123.776) ccw projected
  arc A686 (-155.7825, 124.1629) -> (-155.7904, 123.6745) centre (-148.2041, 123.7947) ccw projected
  arc A687 (-155.4077, 124.3011) -> (-155.7825, 124.1629) centre (-148.5, 105) ccw projected
  arc A688 (-155.0844, 123.9349) -> (-155.4077, 124.3011) centre (-160.9312, 119.0994) ccw projected
  arc A689 (-154.8425, 123.6234) -> (-155.0844, 123.9349) centre (-160.0222, 119.8512) ccw projected
  arc A690 (-154.6673, 123.3672) -> (-154.8425, 123.6234) centre (-159.1041, 120.5199) ccw projected
  arc A691 (-154.3066, 123.4844) -> (-154.6673, 123.3672) centre (-148.5, 105) ccw projected
  arc A692 (-154.3154, 123.7947) -> (-154.3066, 123.4844) centre (-149.0434, 123.7888) ccw projected
  arc A693 (-154.3028, 124.1889) -> (-154.3154, 123.7947) centre (-147.9076, 123.7875) ccw projected
  arc A694 (-154.2565, 124.6752) -> (-154.3028, 124.1889) centre (-146.7304, 123.7136) ccw projected
  arc A695 (-153.872, 124.7836) -> (-154.2565, 124.6752) centre (-148.5, 105) ccw projected
  arc A696 (-153.5785, 124.3932) -> (-153.872, 124.7836) centre (-159.7867, 120.0313) ccw projected
  arc A697 (-153.3618, 124.0636) -> (-153.5785, 124.3932) centre (-158.8215, 120.7095) ccw projected
  arc A698 (-153.2072, 123.7945) -> (-153.3618, 124.0636) centre (-157.8537, 121.304) ccw projected
  arc A699 (-152.8384, 123.883) -> (-153.2072, 123.7945) centre (-148.5, 105) ccw projected
  arc A700 (-152.8228, 124.193) -> (-152.8384, 123.883) centre (-147.5676, 123.7735) ccw projected
  arc A701 (-152.7793, 124.585) -> (-152.8228, 124.193) centre (-146.4354, 123.6831) ccw projected
  arc A702 (-152.6951, 125.0662) -> (-152.7793, 124.585) centre (-145.2676, 123.517) ccw projected
  arc A703 (-152.3033, 125.1441) -> (-152.6951, 125.0662) centre (-148.5, 105) ccw projected
  arc A704 (-152.0413, 124.7318) -> (-152.3033, 125.1441) centre (-158.5726, 120.8705) ccw projected
  arc A705 (-151.8511, 124.3863) -> (-152.0413, 124.7318) centre (-157.5571, 121.4708) ccw projected
  arc A706 (-151.7181, 124.1059) -> (-151.8511, 124.3863) centre (-156.5457, 121.9876) ccw projected
  arc A707 (-151.3435, 124.1652) -> (-151.7181, 124.1059) centre (-148.5, 105) ccw projected
  arc A708 (-151.3036, 124.473) -> (-151.3435, 124.1652) centre (-146.0975, 123.6425) ccw projected
  arc A709 (-151.2295, 124.8604) -> (-151.3036, 124.473) centre (-144.9759, 123.4635) ccw projected
  arc A710 (-151.1078, 125.3335) -> (-151.2295, 124.8604) centre (-143.8247, 123.2064) ccw projected
  arc A711 (-150.7111, 125.3804) -> (-151.1078, 125.3335) centre (-148.5, 105) ccw projected
  arc A712 (-150.4822, 124.9489) -> (-150.7111, 125.3804) centre (-157.2963, 121.6119) ccw projected
  arc A713 (-150.3197, 124.5895) -> (-150.4822, 124.9489) centre (-156.2369, 122.1307) ccw projected
  arc A714 (-150.2091, 124.2995) -> (-150.3197, 124.5895) centre (-155.1881, 122.5665) ccw projected
  arc A715 (-149.831, 124.3292) -> (-150.2091, 124.2995) centre (-148.5, 105) ccw projected
  arc A716 (-149.7671, 124.633) -> (-149.831, 124.3292) centre (-144.6423, 123.3965) ccw projected
  arc A717 (-149.6629, 125.0133) -> (-149.7671, 124.633) centre (-143.5382, 123.1301) ccw projected
  arc A718 (-149.5044, 125.4754) -> (-149.6629, 125.0133) centre (-142.4106, 122.7834) ccw projected
  arc A719 (-149.1052, 125.4911) -> (-149.5044, 125.4754) centre (-148.5, 105) ccw projected
  arc A720 (-148.9109, 125.0429) -> (-149.1052, 125.4911) centre (-155.9658, 122.2508) ccw projected
  circle A721 centre (-148.5, 105) radius 6
  circle A722 centre (-148.5, 105) radius 18.25
  point P0 (0, 0)
  dimension "d11" = 12
  dimension "d12" = 36.5
  constraints: 2 centre point, 2 coincident
  measures "d11" diameter of A721
  measures "d12" diameter of A722
extrude "押し出し3" cut sketch "スケッチ3" against normal blind 0.75 contours A722